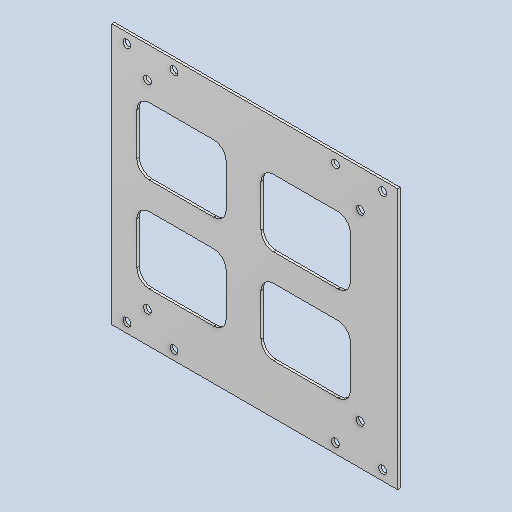
# Autodesk Inventor part: PCB_board_box_buttom
Saved by Autodesk Inventor 2023 (Build 270158000, 158)
## iProperties
Created: 2023-05-25
Part Number: PCB_board_box_buttom
Material: Aluminum
Document SubType Name: Sheet Metal
Designer: 310611102
Density: 2.7 g/cm^3
Sheet Metal Rule: 1mm
Appearance: Satin
Author: 310611102
Autodesk Inventor part; units mm, degrees
ref_plane "YZ Plane" through (0, 0, 0) normal (1, 0, 0) x (0, 1, 0)
ref_plane "XZ Plane" through (0, 0, 0) normal (0, 1, 0) x (-1, 0, 0)
ref_plane "XY Plane" through (0, 0, 0) normal (0, 0, 1) x (1, 0, 0)
sketch "Sketch1" plane through (0, 0, 0) normal (0, 0, 1) x (1, 0, 0)
  line L0 (-57.5, 52.5) -> (57.5, 52.5)
  line L1 (57.5, 52.5) -> (57.5, -52.5)
  line L2 (57.5, -52.5) -> (-57.5, -52.5)
  line L3 (-57.5, -52.5) -> (-57.5, 52.5)
  line L4 (-57.5, 52.5) -> (57.5, -52.5) construction
  line L5 (57.5, 52.5) -> (-57.5, -52.5) construction
  circle A0 centre (42.5, 37.5) radius 1.6
  line L6 (-42.5, 32.5) -> (-16.5, 32.5)
  line L7 (-11.5, 27.5) -> (-11.5, 10.5)
  line L8 (-16.5, 5.5) -> (-42.5, 5.5)
  line L9 (-47.5, 10.5) -> (-47.5, 27.5)
  arc A1 (-42.5, 32.5) -> (-47.5, 27.5) centre (-42.5, 27.5) ccw
  arc A2 (-11.5, 27.5) -> (-16.5, 32.5) centre (-16.5, 27.5) ccw
  arc A3 (-16.5, 5.5) -> (-11.5, 10.5) centre (-16.5, 10.5) ccw
  arc A4 (-47.5, 10.5) -> (-42.5, 5.5) centre (-42.5, 10.5) ccw
  line L10 (38.5, 27.5) -> (38.5, 10.5)
  arc A5 (38.5, 27.5) -> (33.5, 32.5) centre (33.5, 27.5) ccw
  line L11 (7.5, 32.5) -> (33.5, 32.5)
  arc A6 (7.5, 32.5) -> (2.5, 27.5) centre (7.5, 27.5) ccw
  line L12 (2.5, 10.5) -> (2.5, 27.5)
  arc A7 (2.5, 10.5) -> (7.5, 5.5) centre (7.5, 10.5) ccw
  line L13 (33.5, 5.5) -> (7.5, 5.5)
  arc A8 (33.5, 5.5) -> (38.5, 10.5) centre (33.5, 10.5) ccw
  line L14 (-11.5, -10.5) -> (-11.5, -27.5)
  arc A9 (-11.5, -10.5) -> (-16.5, -5.5) centre (-16.5, -10.5) ccw
  line L15 (-42.5, -5.5) -> (-16.5, -5.5)
  arc A10 (-42.5, -5.5) -> (-47.5, -10.5) centre (-42.5, -10.5) ccw
  line L16 (-47.5, -27.5) -> (-47.5, -10.5)
  arc A11 (-47.5, -27.5) -> (-42.5, -32.5) centre (-42.5, -27.5) ccw
  line L17 (-16.5, -32.5) -> (-42.5, -32.5)
  arc A12 (-16.5, -32.5) -> (-11.5, -27.5) centre (-16.5, -27.5) ccw
  line L18 (38.5, -10.5) -> (38.5, -27.5)
  arc A13 (38.5, -10.5) -> (33.5, -5.5) centre (33.5, -10.5) ccw
  line L19 (7.5, -5.5) -> (33.5, -5.5)
  arc A14 (7.5, -5.5) -> (2.5, -10.5) centre (7.5, -10.5) ccw
  line L20 (2.5, -27.5) -> (2.5, -10.5)
  arc A15 (2.5, -27.5) -> (7.5, -32.5) centre (7.5, -27.5) ccw
  line L21 (33.5, -32.5) -> (7.5, -32.5)
  arc A16 (33.5, -32.5) -> (38.5, -27.5) centre (33.5, -27.5) ccw
  circle A17 centre (-43.225, 40.04) radius 1.6
  circle A18 centre (42.5, -36.16) radius 1.6
  circle A19 centre (-43.225, -39.97) radius 1.6
  circle A20 centre (-51.5, 48.5) radius 1.6
  circle A21 centre (-32.5, 48.6) radius 1.6
  line L22 (0, 0) -> (12.5, 0)
  circle A22 centre (-32.5, -48.6) radius 1.6
  circle A23 centre (-51.5, -48.5) radius 1.6
  circle A24 centre (51.5, 48.5) radius 1.6
  circle A25 centre (51.5, -48.5) radius 1.6
  line L23 (0, 0) -> (0, 10.1382)
  circle A26 centre (32.5, 48.6) radius 1.6
  circle A27 centre (32.5, -48.6) radius 1.6
  point P0 (-47.5, 32.5)
  point P1 (-11.5, 5.5)
  point P2 (-11.5, 32.5)
  point P3 (38.5, 32.5)
  point P4 (38.5, 5.5)
  point P5 (2.5, 32.5)
  point P6 (-11.5, -5.5)
  point P7 (-11.5, -32.5)
  point P8 (-47.5, -5.5)
  point P9 (38.5, -5.5)
  point P10 (38.5, -32.5)
  point P11 (2.5, -5.5)
  dimension "d0" = 115
  dimension "d1" = 105
  dimension "d10" = 15
  dimension "d12" = 3.2
  dimension "d13" = 36
  dimension "d14" = 27
  dimension "d15" = 20
  dimension "d16" = 10
  dimension "d17" = 5
  dimension "d20" = 50
  dimension "d23" = 38
  dimension "d38" = 15
  dimension "d39" = 2.54
  dimension "d40" = 3.2
  dimension "d41" = 85.725
  dimension "d42" = 3.2
  dimension "d43" = 3.2
  dimension "d44" = 73.66
  dimension "d45" = 80.01
  dimension "d47" = 3.2
  dimension "d48" = 4
  dimension "d49" = 6
  dimension "d52" = 25
  dimension "d53" = 3.9
  dimension "d54" = 3.2
  dimension "d56" = 97
  dimension "d59" = 3.2
  dimension "d60" = 6
  dimension "d61" = 4
  dimension "d62" = 11
  dimension "d63" = 14
  dimension "d64" = 14.275
  measures "d0" distance of L0.start L0.end
  measures "d1" distance of L0.end L1.end
  measures "d10" distance from line of L0 A0.centre
  measures "d12" diameter of A0
  measures "d13" distance of point (-47.5, 32.5) point (-11.5, 32.5)
  measures "d14" distance of point (-11.5, 32.5) point (-11.5, 5.5)
  measures "d15" distance between parallel lines of L0 L6
  measures "d16" distance between parallel lines of L3 L9
  measures "d17" radius of A1
  measures "d20" distance of L7.start L10.start
  measures "d23" distance of L7.start L14.start
  measures "d38" distance from line of L1 A0.centre
  measures "d39" vertical distance of A0.centre A17.centre
  measures "d40" diameter of A17
  measures "d41" horizontal distance of A0.centre A17.centre
  measures "d42" diameter of A18
  measures "d43" diameter of A19
  measures "d44" distance of A0.centre A18.centre
  measures "d45" distance of A19.centre A17.centre
  measures "d47" diameter of A20
  measures "d48" distance from line of L0 A20.centre
  measures "d49" distance from line of L3 A20.centre
  measures "d52" distance from line of L3 A21.centre
  measures "d53" distance from line of L0 A21.centre
  measures "d54" diameter of A21
  measures "d56" distance of A20.centre A23.centre
  measures "d59" diameter of A24
  measures "d60" distance from line of L1 A24.centre
  measures "d61" distance from line of L0 A24.centre
  measures "d62" distance between parallel lines of L15 L8
  measures "d63" distance between parallel lines of L20 L14
  measures "d64" distance from line of L3 A17.centre
sketch "Sketch2" plane through (0, 0, 1) normal (0, 0, 1) x (1, 0, 0)
  arc A0 (27.5, -15) -> (32.5, -10) centre (27.5, -10) ccw
  line L0 (27.5, -15) -> (7.5, -15)
  arc A1 (2.5, -10) -> (7.5, -15) centre (7.5, -10) ccw
  line L1 (2.5, -10) -> (2.5, 0)
  arc A2 (7.5, 5) -> (2.5, 0) centre (7.5, 0) ccw
  line L2 (7.5, 5) -> (27.5, 5)
  arc A3 (32.5, 0) -> (27.5, 5) centre (27.5, 0) ccw
  line L3 (32.5, 0) -> (32.5, -10)
  arc A4 (-17.5, -15) -> (-12.5, -10) centre (-17.5, -10) ccw
  line L4 (-17.5, -15) -> (-37.5, -15)
  arc A5 (-42.5, -10) -> (-37.5, -15) centre (-37.5, -10) ccw
  line L5 (-42.5, -10) -> (-42.5, 0)
  arc A6 (-37.5, 5) -> (-42.5, 0) centre (-37.5, 0) ccw
  line L6 (-37.5, 5) -> (-17.5, 5)
  arc A7 (-12.5, 0) -> (-17.5, 5) centre (-17.5, 0) ccw
  line L7 (-12.5, 0) -> (-12.5, -10)
  arc A8 (27.5, 20) -> (32.5, 25) centre (27.5, 25) ccw
  line L8 (27.5, 20) -> (7.5, 20)
  arc A9 (2.5, 25) -> (7.5, 20) centre (7.5, 25) ccw
  line L9 (2.5, 25) -> (2.5, 35)
  arc A10 (7.5, 40) -> (2.5, 35) centre (7.5, 35) ccw
  line L10 (7.5, 40) -> (27.5, 40)
  arc A11 (32.5, 35) -> (27.5, 40) centre (27.5, 35) ccw
  line L11 (32.5, 35) -> (32.5, 25)
  arc A12 (-12.5, 35) -> (-17.5, 40) centre (-17.5, 35) ccw
  line L12 (-12.5, 35) -> (-12.5, 25)
  arc A13 (-17.5, 20) -> (-12.5, 25) centre (-17.5, 25) ccw
  line L13 (-17.5, 20) -> (-37.5, 20)
  arc A14 (-42.5, 25) -> (-37.5, 20) centre (-37.5, 25) ccw
  line L14 (-42.5, 25) -> (-42.5, 35)
  arc A15 (-37.5, 40) -> (-42.5, 35) centre (-37.5, 35) ccw
  line L15 (-37.5, 40) -> (-17.5, 40)
  circle A16 centre (42.5, 40) radius 1.6
  line L16 (52.5, 50) -> (52.5, -50)
  line L17 (-52.5, 50) -> (52.5, 50)
  line L18 (-52.5, -50) -> (-52.5, 50)
  line L19 (52.5, -50) -> (-52.5, -50)
  line L20 (62.5, -60) -> (62.5, 60)
  line L21 (62.5, 60) -> (-62.5, 60)
  line L22 (-62.5, 60) -> (-62.5, -60)
  line L23 (-62.5, -60) -> (62.5, -60)
  circle A17 centre (-4.5, 56) radius 1.6
  circle A18 centre (58.5, 12) radius 1.6
  line L24 (-4.5, 12) -> (2.5, 12)
  circle A19 centre (-4.5, -32) radius 1.6
  line L25 (-4.5, 12) -> (-4.5, 17.4476)
  circle A20 centre (-67.5, 12) radius 1.6
  point P0 (57.5, -52.5)
  dimension "d28" = 10
  dimension "d29" = 3.2
  dimension "d30" = 6
  dimension "d31" = 3.2
  dimension "d32" = 6
  measures "d28" distance between parallel lines of L16 L20
  measures "d29" diameter of A17
  measures "d30" distance from line of L17 A17.centre
  measures "d31" diameter of A18
  measures "d32" distance from line of L16 A18.centre
extrude "Plate1" add sketch "Sketch1" along normal blind 1
equation "\"折彎半徑\" = 厚度"
equation "\"折彎離隙寬度\" = 厚度"
equation "\"折彎離隙深度\" = 0.5 * 厚度"
equation "\"轉角離隙大小\" = 4 * 厚度"
equation "\"最小剩餘\" = 2 * 厚度"
equation "\"轉移半徑\" = 折彎半徑"
equation "\"Jacobi半徑大小\" = 折彎半徑"
equation "\"間隙大小\" = 厚度"
body "Solid1"
